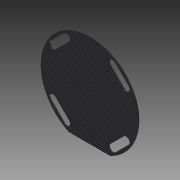
# Autodesk Inventor part: Bottom Plate
Saved by Autodesk Inventor 2015 (Build 190159000, 159)
## iProperties
Created: 2016-08-08
Part Number: Bottom Plate
Material: Generic
Document SubType Name: Modeling
Designer: James Yelland
Density: 1 g/cm^3
Appearance: Default
Author: James Yelland
Autodesk Inventor part; units mm, degrees
ref_plane "YZ Plane" through (0, 0, 0) normal (1, 0, 0) x (0, 1, 0)
ref_plane "XZ Plane" through (0, 0, 0) normal (0, 1, 0) x (-1, 0, 0)
ref_plane "XY Plane" through (0, 0, 0) normal (0, 0, 1) x (1, 0, 0)
sketch "Sketch1" plane through (0, 0, 0) normal (0, 1, 0) x (-1, 0, 0)
  line L0 (-69.2965, -69.2965) -> (-54.4472, -84.1457)
  line L1 (-44.5477, -84.1457) -> (-43.8406, -83.4386)
  line L2 (-43.8406, -73.5391) -> (-73.5391, -43.8406)
  line L3 (-83.4386, -43.8406) -> (-84.1457, -44.5477)
  line L4 (-84.1457, -54.4472) -> (-69.2965, -69.2965)
  arc A0 (-43.8406, -83.4386) -> (-43.8406, -73.5391) centre (-48.7904, -78.4889) ccw
  arc A1 (-54.4472, -84.1457) -> (-44.5477, -84.1457) centre (-49.4975, -79.196) ccw
  arc A2 (-84.1457, -44.5477) -> (-84.1457, -54.4472) centre (-79.196, -49.4975) ccw
  arc A3 (-73.5391, -43.8406) -> (-83.4386, -43.8406) centre (-78.4889, -48.7904) ccw
  line L5 (69.2965, -69.2965) -> (84.1457, -54.4472)
  line L6 (84.1457, -44.5477) -> (83.4386, -43.8406)
  line L7 (73.5391, -43.8406) -> (43.8406, -73.5391)
  line L8 (43.8406, -83.4386) -> (44.5477, -84.1457)
  line L9 (54.4472, -84.1457) -> (69.2965, -69.2965)
  arc A4 (83.4386, -43.8406) -> (73.5391, -43.8406) centre (78.4889, -48.7904) ccw
  arc A5 (84.1457, -54.4472) -> (84.1457, -44.5477) centre (79.196, -49.4975) ccw
  arc A6 (44.5477, -84.1457) -> (54.4472, -84.1457) centre (49.4975, -79.196) ccw
  arc A7 (43.8406, -73.5391) -> (43.8406, -83.4386) centre (48.7904, -78.4889) ccw
  line L10 (69.2965, 69.2965) -> (54.4472, 84.1457)
  line L11 (44.5477, 84.1457) -> (43.8406, 83.4386)
  line L12 (43.8406, 73.5391) -> (73.5391, 43.8406)
  line L13 (83.4386, 43.8406) -> (84.1457, 44.5477)
  line L14 (84.1457, 54.4472) -> (69.2965, 69.2965)
  arc A8 (43.8406, 83.4386) -> (43.8406, 73.5391) centre (48.7904, 78.4889) ccw
  arc A9 (54.4472, 84.1457) -> (44.5477, 84.1457) centre (49.4975, 79.196) ccw
  arc A10 (84.1457, 44.5477) -> (84.1457, 54.4472) centre (79.196, 49.4975) ccw
  arc A11 (73.5391, 43.8406) -> (83.4386, 43.8406) centre (78.4889, 48.7904) ccw
  line L15 (-69.2965, 69.2965) -> (-84.1457, 54.4472)
  line L16 (-84.1457, 44.5477) -> (-83.4386, 43.8406)
  line L17 (-73.5391, 43.8406) -> (-43.8406, 73.5391)
  line L18 (-43.8406, 83.4386) -> (-44.5477, 84.1457)
  line L19 (-54.4472, 84.1457) -> (-69.2965, 69.2965)
  arc A12 (-83.4386, 43.8406) -> (-73.5391, 43.8406) centre (-78.4889, 48.7904) ccw
  arc A13 (-84.1457, 54.4472) -> (-84.1457, 44.5477) centre (-79.196, 49.4975) ccw
  arc A14 (-44.5477, 84.1457) -> (-54.4472, 84.1457) centre (-49.4975, 79.196) ccw
  arc A15 (-43.8406, 73.5391) -> (-43.8406, 83.4386) centre (-48.7904, 78.4889) ccw
  line L20 (0, 0) -> (44.3749, -95.1623)
  line L21 (0, 0) -> (105, 0) construction
  line L22 (0, 0) -> (-44.3749, -95.1623)
  line L23 (0, 0) -> (105, 0) construction
  line L24 (-44.3749, -95.1623) -> (44.3749, -95.1623)
  arc A16 (44.3749, -95.1623) -> (-44.3749, -95.1623) centre (0, 0) ccw
  line L25 (0, 0) -> (-58.6899, 58.6899)
  line L26 (0, 0) -> (58.6899, 58.6899)
  line L27 (0, 0) -> (58.6899, -58.6899)
  line L28 (0, 0) -> (-58.6899, -58.6899)
  point P0 (-49.4975, -89.0955)
  point P1 (-38.8909, -78.4889)
  point P2 (-78.4889, -38.8909)
  point P3 (-89.0955, -49.4975)
  point P4 (89.0955, -49.4975)
  point P5 (78.4889, -38.8909)
  point P6 (38.8909, -78.4889)
  point P7 (49.4975, -89.0955)
  point P8 (49.4975, 89.0955)
  point P9 (38.8909, 78.4889)
  point P10 (78.4889, 38.8909)
  point P11 (89.0955, 49.4975)
  point P12 (-89.0955, 49.4975)
  point P13 (-78.4889, 38.8909)
  point P14 (-38.8909, 78.4889)
  point P15 (-49.4975, 89.0955)
  dimension "d6" = 28
  dimension "d8" = 15
  dimension "d9" = 56
  dimension "d10" = 7
  dimension "d13" = 360
  dimension "d15" = 65
  dimension "d16" = 115
  constraints: 58 end point, 37 point on line, 34 point on circle, 17 centre point, 8 tangent, 4 midpoint, 4 perpendicular, 3 coincident, 3 equal radius, 2 equal length, 2 horizontal, 107 other
  measures "d6" distance of L0.start point (-49.497, -89.095)
  measures "d8" distance of point (-49.497, -89.095) point (-38.891, -78.489)
  measures "d9" distance of point (-38.891, -78.489) point (-78.489, -38.891)
  measures "d10" radius of A0
  measures "d15" angle of L20 L21
  measures "d16" angle of L22 L23
extrude "Extrusion1" add sketch "Sketch1" along normal blind 2
body "Solid1"
